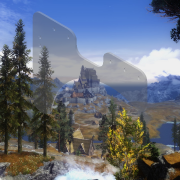
# Autodesk Inventor part: C13_TK_UpperFrameSupportWheel
Saved by Autodesk Inventor 2015 SP1 (Build 190203100, 203)
## iProperties
Created: 2016-01-16
Part Number: C13_TK_UpperFrameSupportWheel
Material: Polycarbonate, Clear
Document SubType Name: Modeling
Designer: TheeTimatahee
Density: 1.2 g/cm^3
Appearance: Polycarbonate - Clear
Mass: 55.1739 g
Surface Area: 316.631 cm^2
Volume: 45.9783 cm^3
Author: TheeTimatahee
Autodesk Inventor part; units mm, degrees
ref_plane "YZ Plane" through (0, 0, 0) normal (1, 0, 0) x (0, 1, 0)
ref_plane "XZ Plane" through (0, 0, 0) normal (0, 1, 0) x (-1, 0, 0)
ref_plane "XY Plane" through (0, 0, 0) normal (0, 0, 1) x (1, 0, 0)
sketch "Sketch1" plane through (0, 0, 0) normal (0, 0, 1) x (1, 0, 0)
  line L0 (-101.6, -76.2) -> (101.6, -76.2)
  line L1 (101.6, -76.2) -> (101.6, 76.2)
  line L2 (101.6, 76.2) -> (-101.6, 76.2)
  line L3 (-101.6, 76.2) -> (-101.6, -76.2)
  line L4 (-101.6, -76.2) -> (101.6, 76.2) construction
  line L5 (101.6, -76.2) -> (-101.6, 76.2) construction
  point P0 (0, 0)
  dimension "d0" = 152.4
  dimension "d1" = 203.2
  constraints: 12 end point, 2 midpoint, 2 parallel, 1 horizontal, 1 perpendicular
  measures "d0" distance of L0.end L1.end
  measures "d1" distance of L1.end L2.end
extrude "Extrusion1" add sketch "Sketch1" along normal blind 3.175
sketch "Sketch2" plane through (0, 0, 0) normal (0, 0, -1) x (-1, 0, 0)
  circle A0 centre (-37.1038, -82.4738) radius 101.092
  circle A1 centre (-37.1038, -82.4738) radius 107.442
  line L0 (-101.6, -76.2) -> (-101.6, 76.2) projected
  line L1 (-101.6, 3.4565) -> (-101.6, -76.2)
  line L2 (-101.6, -76.2) -> (70.1549, -76.2)
  line L3 (101.6, -76.2) -> (-101.6, -76.2) projected
  point P0 (0, 0)
  dimension "d4" = 214.884
  constraints: 4 end point, 2 centre point, 2 point on circle, 2 point on line, 1 coincident, 1 vertical, 2 other
  measures "d4" diameter of A1
extrude "Extrusion2" cut sketch "Sketch2" against normal blind 25.4 contours L2 L0 A0 | A0 L0 A1 L2 picked at (8.0579, -71.6086) picked at (67.4292, -71.4153)
fillet "Fillet1" radius 12.7 5 edges at (101.6, 76.2, 1.5875) (-101.6, 76.2, 1.5875) (-101.6, -76.2, 1.5875) (-70.1549, -76.2, 1.5875) (101.6, 3.4565, 1.5875)
sketch "Sketch3" plane through (0, 0, 0) normal (0, 0, -1) x (-1, 0, 0)
  line L0 (76.2027, 73.1012) -> (-660.4, 73.1012) projected
  line L1 (-660.4, 53.8988) -> (76.2027, 53.8988) projected
  circle A0 centre (-647.7, 63.5) radius 2.0701 projected
  circle A1 centre (-622.3, 63.5) radius 2.0701 projected
  circle A2 centre (-596.9, 63.5) radius 2.0701 projected
  circle A3 centre (-571.5, 63.5) radius 2.0701 projected
  circle A4 centre (-546.1, 63.5) radius 2.0701 projected
  circle A5 centre (-520.7, 63.5) radius 2.0701 projected
  circle A6 centre (-495.3, 63.5) radius 2.0701 projected
  circle A7 centre (-469.9, 63.5) radius 2.0701 projected
  circle A8 centre (-444.5, 63.5) radius 2.0701 projected
  circle A9 centre (-419.1, 63.5) radius 2.0701 projected
  circle A10 centre (-393.7, 63.5) radius 2.0701 projected
  circle A11 centre (-368.3, 63.5) radius 2.0701 projected
  circle A12 centre (-342.9, 63.5) radius 2.0701 projected
  circle A13 centre (-317.5, 63.5) radius 2.0701 projected
  circle A14 centre (-292.1, 63.5) radius 2.0701 projected
  circle A15 centre (-266.7, 63.5) radius 2.0701 projected
  circle A16 centre (-241.3, 63.5) radius 2.0701 projected
  circle A17 centre (-215.9, 63.5) radius 2.0701 projected
  circle A18 centre (-190.5, 63.5) radius 2.0701 projected
  circle A19 centre (-165.1, 63.5) radius 2.0701 projected
  circle A20 centre (-139.7, 63.5) radius 2.0701 projected
  circle A21 centre (-114.3, 63.5) radius 2.0701 projected
  circle A22 centre (-88.9, 63.5) radius 2.0701 projected
  circle A23 centre (-63.5, 63.5) radius 2.0701 projected
  circle A24 centre (-38.1, 63.5) radius 2.0701 projected
  circle A25 centre (-12.7, 63.5) radius 2.0701 projected
  circle A26 centre (12.7, 63.5) radius 2.0701 projected
  circle A27 centre (38.1, 63.5) radius 2.0701 projected
  circle A28 centre (63.5, 63.5) radius 2.0701 projected
  line L2 (97.2058, -44.2468) -> (78.359, -44.2468) projected
  line L3 (78.359, -44.2468) -> (76.2, -42.0878) projected
  line L4 (76.2, 16.8402) -> (76.2, -42.0878) projected
  line L5 (76.2, 16.8402) -> (78.359, 18.9992) projected
  line L6 (97.2058, 18.9992) -> (78.359, 18.9992) projected
  line L7 (97.2058, -44.2468) -> (97.2058, 18.9992) projected
  circle A29 centre (88.9, 12.7762) radius 2.0701 projected
  circle A30 centre (88.9, 0.0762) radius 2.0701 projected
  circle A31 centre (88.9, -12.6238) radius 2.0701 projected
  circle A32 centre (88.9, -25.3238) radius 2.0701 projected
  circle A33 centre (88.9, -38.0238) radius 2.0701 projected
  line L8 (76.2027, 73.1012) -> (76.2027, 53.8988) projected
  line L9 (-660.4, 53.8988) -> (-660.4, 73.1012) projected
  point P0 (0, 0)
  point P1 (88.9, 25.4762)
  point P2 (88.9, 38.1762)
  dimension "d17" = 12.7
  constraints: 1 coincident, 1 vertical, 2 other
  measures "d17" distance of point (88.9, 12.776) point (88.9, 25.476)
hole "Hole1" at (88.9, 63.5, 0) at (63.5, 63.5, 0) at (38.1, 63.5, 0) at (12.7, 63.5, 0) at (-12.7, 63.5, 0) at (-38.1, 63.5, 0) at (-63.5, 63.5, 0) at (-88.9, 12.7762, 0) at (-88.9, 0.0762, 0) at (-88.9, -12.6238, 0) at (-88.9, -25.3238, 0) at (-88.9, -38.0238, 0) at (-88.9, 25.4762, 0) at (-88.9, 38.1762, 0) direction (0, 0, 1) diameter 4.1402 end through all
sketch "Sketch4" plane through (0, 0, 0) normal (0, 0, -1) x (-1, 0, 0)
  line L0 (-88.9, 76.2) -> (88.9, 76.2) projected
  line L1 (-25.4, 76.2) -> (25.4, 76.2)
  line L2 (25.4, 76.2) -> (25.4, 44.45)
  line L3 (25.4, 44.45) -> (-25.4, 44.45)
  line L4 (-25.4, 44.45) -> (-25.4, 76.2)
  line L5 (-101.6, 25.9294) -> (-101.6, 63.5) projected
  point P0 (0, 0)
  dimension "d23" = 31.75
  dimension "d24" = 50.8
  dimension "d25" = 76.2
  constraints: 8 end point, 2 parallel, 1 horizontal, 1 perpendicular, 1 point on line
  measures "d23" distance of L3.end L1.start
  measures "d24" distance of L2.end L3.end
  measures "d25" distance between parallel lines of L5 L4
extrude "Extrusion3" cut sketch "Sketch4" against normal through all
fillet "Fillet2" radius 12.7 4 edges at (25.4, 76.2, 1.5875) (25.4, 44.45, 1.5875) (-25.4, 44.45, 1.5875) (-25.4, 76.2, 1.5875)
body "Solid1"
